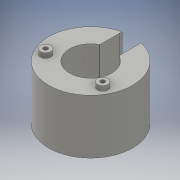
# Autodesk Inventor part: motor-mount
Saved by Autodesk Inventor 2016 (Build 200138000, 138)
## iProperties
Created: 2016-10-30
Part Number: motor-mount
Material: Generic
Document SubType Name: Modeling
Designer: Matt Ruffner
Density: 1 g/cm^3
Appearance: Default
Author: Matt Ruffner
Autodesk Inventor part; units mm, degrees
ref_plane "YZ Plane" through (0, 0, 0) normal (1, 0, 0) x (0, 1, 0)
ref_plane "XZ Plane" through (0, 0, 0) normal (0, 1, 0) x (-1, 0, 0)
ref_plane "XY Plane" through (0, 0, 0) normal (0, 0, 1) x (1, 0, 0)
sketch "Sketch1" plane through (0, 0, 0) normal (0, 1, 0) x (-1, 0, 0)
  circle A0 centre (0, 0) radius 22
  dimension "d0" = 44
  constraints: 1 centre point, 1 coincident
  measures "d0" diameter of A0
extrude "Extrusion1" add sketch "Sketch1" along normal blind 25.5
sketch "Sketch2" plane through (0, 25.5, 0) normal (0, 1, 0) x (1, 0, 0)
  arc A0 (-9.696, -5.3) -> (-9.696, 5.3) centre (0, 0) ccw
  circle A1 centre (0, 0) radius 22 projected
  line L0 (-9.696, -5.3) -> (-21.352, -5.3)
  line L1 (-9.696, 5.3) -> (-21.352, 5.3)
  point P0 (-11.05, 0)
  dimension "d4" = 22.1
  constraints: 4 end point, 4 point on circle, 1 centre point, 1 coincident, 1 horizontal
  measures "d4" diameter of A0
extrude "Extrusion2" cut sketch "Sketch2" against normal blind 25.5 contours L0 A1 L1 A0 picked at (0.8234, -1.0096)
sketch "Sketch3" plane through (0, 25.5, 0) normal (0, 1, 0) x (1, 0, 0)
  circle A0 centre (-17.25, 0) radius 2.75
  arc A1 (-21.352, -5.3) -> (-21.352, 5.3) centre (0, 0) ccw projected
  circle A2 centre (0, 0) radius 22
  circle A3 centre (-17.25, 0) radius 1.125
  circle A4 centre (8.625, -14.9389) radius 2.75
  circle A5 centre (8.625, -14.9389) radius 1.125
  circle A6 centre (8.625, 14.9389) radius 2.75
  circle A7 centre (8.625, 14.9389) radius 1.125
  dimension "d9" = 5.5
  dimension "d10" = 2
  dimension "d11" = 2.25
  dimension "d14" = 360
  constraints: 6 centre point, 4 coincident, 16 other
  measures "d9" diameter of A0
  measures "d11" diameter of A3
extrude "Extrusion3" cut sketch "Sketch3" against normal blind 10 contours A5 | A7
sketch "Sketch4" plane through (0, 25.5, 0) normal (0, 1, 0) x (1, 0, 0)
  circle A0 centre (8.625, -14.9389) radius 1.125 projected
  circle A1 centre (8.625, 14.9389) radius 1.125 projected
  circle A2 centre (8.625, -14.9389) radius 2.75
  circle A3 centre (8.625, 14.9389) radius 2.75
  point P0 (0, 0)
  dimension "d18" = 5.5
  dimension "d19" = 5.5
  constraints: 2 centre point, 2 coincident
  measures "d18" diameter of A2
  measures "d19" diameter of A3
extrude "Extrusion4" add sketch "Sketch4" along normal blind 2.5
sketch "Sketch5" plane through (0, 0, 0) normal (0, -1, 0) x (1, 0, 0)
  line L0 (-9.696, -5.3) -> (-21.352, -5.3) projected
  arc A0 (-21.352, -5.3) -> (-21.352, 5.3) centre (0, 0) ccw projected
  line L1 (-21.352, 5.3) -> (-9.696, 5.3) projected
  arc A1 (-9.696, -5.3) -> (-9.696, 5.3) centre (0, 0) ccw projected
  line L2 (-21.352, -5.3) -> (-21.352, -3.3)
  line L3 (-21.352, -3.3) -> (-10.5457, -3.3)
  line L4 (-10.5457, -3.3) -> (-10.5457, -5.3)
  line L5 (-21.352, 5.3) -> (-21.352, 3.3)
  line L6 (-21.352, 3.3) -> (-10.5457, 3.3)
  line L7 (-10.5457, 3.3) -> (-10.5457, 5.3)
  dimension "d22" = 2
  dimension "d23" = 2
  constraints: 12 end point, 5 point on line, 3 perpendicular, 1 vertical
  measures "d22" distance of L0.end L2.end
  measures "d23" distance of L1.start L5.end
extrude "Extrusion5" add sketch "Sketch5" along normal blind 3
chamfer "Chamfer1" distance 1 angle 45 1 edges at (-15.9489, 0, 3.3)
chamfer "Chamfer2" distance 1 angle 45 3 edges at (-15.9489, 0, -3.3) (-15.9489, 0, 5.3) (-15.9489, 0, -5.3)
sketch "Sketch6" plane through (0, 25.5, 0) normal (0, 1, 0) x (1, 0, 0)
  line L0 (-21.352, -5.3) -> (-21.352, -4.8)
  line L1 (-21.352, -5.3) -> (-21.352, -3.3) projected
  line L2 (-21.352, -4.8) -> (-19.9573, -5.05)
  line L3 (-19.9573, -5.05) -> (-9.8667, -5.05)
  line L4 (-9.8667, -5.05) -> (-9.696, -5.3)
  line L5 (-9.696, -5.3) -> (-21.352, -5.3) projected
  line L6 (-9.696, -5.3) -> (-21.352, -5.3)
  line L7 (-22.4952, 0) -> (-9.696, 0)
  line L8 (-21.352, 5.3) -> (-21.352, 4.8)
  line L9 (-21.352, 4.8) -> (-19.9573, 5.05)
  line L10 (-19.9573, 5.05) -> (-9.8667, 5.05)
  line L11 (-9.8667, 5.05) -> (-9.696, 5.3)
  line L12 (-9.696, 5.3) -> (-21.352, 5.3)
  point P0 (0, 0)
  dimension "d32" = 0.5
  constraints: 22 end point, 5 symmetric about line, 1 horizontal, 1 parallel, 1 perpendicular, 1 point on line
  measures "d32" distance of L0.start L0.end
extrude "Extrusion6" add sketch "Sketch6" against normal up to surface (28.5 mm away)
body "Solid1"
